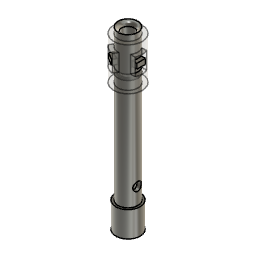
RETHI Vacuum Chamber (Autodesk Fusion 360 design; units mm, degrees)
Autodesk Fusion 360 part; units mm, degrees
sketch "Sketch1" plane through (0, 0, 0) normal (0, 0, 1) x (1, 0, 0)
  circle A0 centre (0, 0) radius 4.445
  circle A1 centre (0, 0) radius 6.35
  circle A2 centre (0, 0) radius 2.8575
  dimension "chamberTrack" = 8.89
  dimension "d2" = 12.7
  dimension "chamberDiam" = 5.715
  constraint coincident A0.centre A1.centre
  constraint concentric A0 A2
  measures "chamberTrack" diameter of A0
  measures "d2" diameter of A1
  measures "chamberDiam" diameter of A2
extrude "Extrude1" add sketch "Sketch1" against normal blind 2.54 contours A0 makes body 1
extrude "Extrude2" add sketch "Sketch1" against normal blind 7.62 contours A1 bodies 1
extrude "Extrude3" add sketch "Sketch1" along normal blind 53.34 contours A0 bodies 1
ref_plane "WorkPlane1" through (4.445, 0, 87.4605) normal (1, 0, 0) x (0, -1, 0)
sketch "Sketch2" plane through (4.445, 0, 87.4605) normal (1, 0, 0) x (0, 1, 0)
  circle A0 centre (0, -76.2) radius 1.905
  dimension "d15" = 3.81
  measures "d15" diameter of A0
extrude "Extrude4" cut sketch "Sketch2" against normal blind 2.54 bodies 1
ref_plane "WorkPlane2" through (0, 0, 48.26) normal (0, 0, 1) x (1, 0, 0)
ref_plane "WorkPlane1" through (0, 0, 49.53) normal (0, 0, 1) x (1, 0, 0) in component "Component"
sketch "Sketch1 (2)" plane through (0, 0, 49.53) normal (0, 0, 1) x (1, 0, 0) in component "Component"
  circle A0 centre (0, 0) radius 4.445
  circle A1 centre (0, 0) radius 6.35
  circle A2 centre (0, 0) radius 4.445
  circle A3 centre (0, 0) radius 4.445
  constraint concentric A0 A2
  constraint concentric A1 A3
extrude "Extrude1'" add sketch "Sketch1 (2)" along normal blind 19.05 separate body makes body 2 in component "Component"
ref_plane "WorkPlane2" through (6.35, 0, 63.864) normal (1, 0, 0) x (0, -1, 0) in component "Component"
sketch "Sketch2 (2)" plane through (6.35, 0, 62.594) normal (1, 0, 0) x (0, 1, 0) in component "Component"
  line L0 (-2.54, 0.906) -> (2.54, 0.906)
  line L1 (2.54, 0.906) -> (2.54, -6.714)
  line L2 (2.54, -6.714) -> (-2.54, -6.714)
  line L3 (-2.54, -6.714) -> (-2.54, 0.906)
  line L4 (6.35, 5.986) -> (-6.35, 5.986)
  line L5 (6.35, -13.064) -> (-6.35, -13.064)
  dimension "compressionRoom" = 7.62
  dimension "d74" = 6.35
  constraint horizontal L0
  constraint vertical L1
  constraint horizontal L2
  constraint vertical L3
  measures "compressionRoom" distance of L0.start L2.end
  measures "d74" distance of L2 L5
extrude "Extrude2'" cut sketch "Sketch2 (2)" along normal up to surface end surface at (4.4229, -0.4426, 62.23) on bodies 2 bodies 2 in component "Component"
pattern_circular "C-Pattern1" count 3 over 360 about axis through (0, 0, 68.58) along (0, 0, -1) of 4 faces at (5.0958, 2.54, 60.96) (5.3616, 1.9489, 55.88) (5.0958, -2.54, 58.42) (5.3616, 1.9489, 63.5) on bodies 2 in component "Component"
sketch "Sketch3" plane through (0, 0, 53.34) normal (0, 0, 1) x (-1, 0, 0) in component "Component"
  circle A0 centre (0, 0) radius 2.8575
  circle A1 centre (0, 0) radius 4.445
  circle A2 centre (0, 0) radius 3.4078
  circle A3 centre (0, 0) radius 3.776
  point P0 (-0.3758, -4.4291)
  point P1 (-3.6478, -2.54)
  constraint concentric A0 A2
  constraint coincident A0.centre A1.centre
ref_plane "WorkPlane1" through (-2.6441, -4.5796, 61.595) normal (0, 0, -1) x (-0.866025, 0.5, 0) in component "Component'"
sketch "Sketch1 (3)" plane through (-2.6441, -4.5796, 61.595) normal (0, 0, -1) x (1, 0, 0) in component "Component'"
  circle A0 centre (2.6441, -4.5796) radius 2.8575
  circle A1 centre (2.6441, -4.5796) radius 4.445
  circle A2 centre (2.6441, -4.5796) radius 2.8575
  circle A3 centre (2.6441, -4.5796) radius 4.3839
  constraint concentric A0 A2
  constraint concentric A2 A3
extrude "Extrude1''" add sketch "Sketch1 (3)" against normal blind 14.605 separate body contours A3 makes body 3 in component "Component'"
ref_plane "WorkPlane2" through (4.3839, 0, 66.7779) normal (1, 0, 0) x (0, -1, 0) in component "Component'"
extrude "Extrude3'" add 1 faces at (3.8482, 0.3598, 61.595) along direction (0, 0, -1) blind 0.762 on bodies 3 bodies 3 in component "Component'"
sketch "Sketch2 (3)" plane through (4.3839, 0, 64.7583) normal (1, 0, 0) x (0, 1, 0) in component "Component'"
  line L0 (-2.032, -1.27) -> (2.032, -1.27)
  line L1 (2.032, -1.27) -> (2.032, 1.27)
  line L2 (2.032, 1.27) -> (-2.032, 1.27)
  line L3 (-2.032, 1.27) -> (-2.032, -1.27)
  dimension "d72" = 2.54
  constraint horizontal L0
  constraint vertical L1
  constraint horizontal L2
  constraint vertical L3
  measures "d72" distance of L0.end L1.end
extrude "Extrude2''" cut sketch "Sketch2 (3)" against normal blind 1.016 bodies 3 in component "Component'"
pattern_circular "C-Pattern1'" count 3 over 360 about axis through (0, 0, 76.2) along (0, 0, -1) of 4 faces at (3.7066, 0, 66.0283) (3.5401, -2.032, 64.3349) (3.5401, 2.032, 65.1816) (3.7066, 0, 63.4883) on bodies 3 in component "Component'"
sketch "Sketch1 (4)" plane through (3.3679, 0, 2.54) normal (1, 0, 0) x (0, 1, 0) in component "Component''"
  line L0 (-2.032, 66.0283) -> (-2.032, 63.4883)
  line L1 (2.032, 63.4883) -> (2.032, 66.0283)
  line L2 (2.032, 66.0283) -> (-2.032, 66.0283)
  line L3 (-1.905, 65.913) -> (1.905, 65.913)
  line L4 (1.905, 65.913) -> (1.905, 63.5918)
  line L5 (1.905, 63.5918) -> (-1.905, 63.5918)
  line L6 (-1.905, 63.5918) -> (-1.905, 65.913)
  line L7 (-2.032, 63.4883) -> (2.032, 63.4883)
  constraint horizontal L3
  constraint vertical L4
  constraint horizontal L5
  constraint vertical L6
extrude "Extrude1'''" add sketch "Sketch1 (4)" along normal blind 2.54 separate body contours L3 L4 L5 L6 makes body 4 in component "Component''"
pattern_circular "C-Pattern1''" count 3 over 360 about axis through (0, 0, 76.2) along (0, 0, -1) of bodies 4 makes body 5 at (-2.6572, -3.3324, 68.453) makes body 6 at (-3.0806, 4.0657, 68.453) in component "Component''"
fillet "Fillet1" radius 1.905 1 edges at (-2.6641, 1.0333, 76.2) on bodies 3 in component "Component'"
sketch "Sketch4" plane through (0, 0, -2.54) normal (0, 0, -1) x (1, 0, 0)
  circle A0 centre (0, 0) radius 2.8575
  circle A1 centre (0, 0) radius 4.445
  circle A2 centre (0, 0) radius 6.35
  circle A3 centre (0, 0) radius 4.445
  constraint coincident A0.centre A1.centre
  constraint concentric A2 A3
extrude "Extrude6" cut sketch "Sketch4" along normal blind 7.62 and the other way blind 2.54 contours A2 bodies 1
sketch "Sketch5" plane through (0, 0, -2.54) normal (0, 0, -1) x (1, 0, 0)
  circle A0 centre (0, 0) radius 2.8575
  circle A1 centre (0, 0) radius 4.445
  circle A2 centre (0, 0) radius 5.4229
  circle A3 centre (0, 0) radius 5.4229
  circle A4 centre (0, 0) radius 2.8575
  dimension "bearingInner" = 10.8458
  constraint coincident A0.centre A1.centre
  constraint concentric A3 A4
  measures "bearingInner" diameter of A2
extrude "Extrude7" add sketch "Sketch5" against normal blind 6.35 contours A2 A3 bodies 1
extrude "Extrude8" add 1 faces at (4.5369, 0.4114, -2.54) along direction (0, 0, -1) blind 5.08 on bodies 1 bodies 1
move_body "Move1" bodies 3 to x (1, 0, 0) y (0, 1, 0) z (0, 0, 1) at (0, 0, -7.62) in component "Component'"
move_body "Move1'" bodies 4 5 6 to x (1, 0, 0) y (0, 1, 0) z (0, 0, 1) at (0, 0, -7.62) in component "Component''"
sketch "Sketch6" plane through (0, 0, 53.34) normal (0, 0, 1) x (-1, 0, 0)
  circle A0 centre (0, 0) radius 2.8575
  circle A1 centre (0, 0) radius 4.445
  circle A2 centre (0, 0) radius 3.4737
  circle A3 centre (0, 0) radius 3.8771
  dimension "lipIn" = 6.9473
  dimension "lipOut" = 7.7543
  constraint concentric A0 A2
  constraint concentric A0 A3
  measures "lipIn" diameter of A2
  measures "lipOut" diameter of A3
extrude "Extrude9" cut sketch "Sketch6" against normal blind 1.27 contours A3 bodies 1
sketch "Sketch7" plane through (0, 0, 55.753) normal (0, 0, -1) x (1, 0, 0)
  circle A0 centre (0, 0) radius 2.8575
  circle A1 centre (0, 0) radius 4.3839
  circle A2 centre (0, 0) radius 3.4737
  circle A3 centre (0, 0) radius 3.8771
  dimension "d88" = 6.9473
  dimension "d89" = 7.7543
  constraint concentric A0 A2
  constraint coincident A0.centre A1.centre
  measures "d88" diameter of A2
  measures "d89" diameter of A3
extrude "Extrude4'" cut sketch "Sketch7" against normal blind 1.27 contours A3 sketch seen with x (1, 0, 0) y (0, 1, 0) z (0, 0, 1) at (0, 0, -2.54) bodies 3 in component "Component'"
component "Component" placed x (1, 0, 0) y (0, 1, 0) z (0, 0, 1) at (0, 0, 0)
component "Component'" placed x (1, 0, 0) y (0, 1, 0) z (0, 0, 1) at (0, 0, 2.54)
component "Component''" placed x (1, 0, 0) y (0, 1, 0) z (0, 0, 1) at (0, 0, 0)
equation "d2 = chamberTrack + 0.15 in"
equation "chamberDiam = hexDiam + 0.1 in"
equation "hexDiam = 0.125 in"
equation "length = armLength - 1.9 in"
equation "armLength = 4 in"
equation "d88 = lipIn"
equation "d89 = lipOut"
